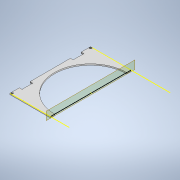
# Autodesk Inventor part: Box_Walls_2
Saved by Autodesk Inventor 2022 (Build 260153000, 153)
## iProperties
Created: 2023-02-27
Part Number: Box_Walls_2
Material: Generic
Document SubType Name: Modeling
Designer: zarek
Density: 1 g/cm^3
Appearance: Default
Author: zarek
Autodesk Inventor part; units mm, degrees
ref_plane "YZ Plane" through (0, 0, 0) normal (1, 0, 0) x (0, 1, 0)
ref_plane "XZ Plane" through (0, 0, 0) normal (0, 1, 0) x (-1, 0, 0)
ref_plane "XY Plane" through (0, 0, 0) normal (0, 0, 1) x (1, 0, 0)
sketch "Sketch1" plane through (0, 0, 0) normal (0, 1, 0) x (-1, 0, 0)
  line L0 (101.6, -101.6) -> (-101.6, -101.6)
  line L1 (-101.6, -101.6) -> (-101.6, 101.6)
  line L2 (-101.6, 101.6) -> (101.6, 101.6)
  line L3 (101.6, 101.6) -> (101.6, -101.6)
  line L4 (96.6, -96.6) -> (-96.6, -96.6)
  line L5 (-96.6, -96.6) -> (-96.6, 96.6)
  line L6 (-96.6, 96.6) -> (96.6, 96.6)
  line L7 (96.6, 96.6) -> (96.6, -96.6)
  line L8 (101.6, 101.6) -> (-40.4, 101.6)
  circle A0 centre (0, 0) radius 86.4
  circle A1 centre (0, 0) radius 109.3376
  line L9 (-40.4, 101.6) -> (-101.6, 40.4)
  line L10 (-45.4, 101.6) -> (-101.6, 45.4)
  line L11 (96.6, 96.6) -> (96.6, 101.6)
  line L12 (-45.4, 101.6) -> (-35.4, 101.6)
  line L13 (-35.4, 101.6) -> (-35.4, 96.6)
  line L14 (-35.4, 96.6) -> (-45.4, 96.6)
  line L15 (-45.4, 96.6) -> (-45.4, 101.6)
  circle A2 centre (0, 0) radius 111.3376
  point P0 (96.6, 51.2168)
  point P1 (101.6, 40.4)
  point P2 (101.6, -40.4)
  point P3 (96.6, -51.2168)
  point P4 (-96.6, 45.4)
  point P5 (-45.4, 96.6)
  dimension "d0" = 203.2
  dimension "d1" = 203.2
  dimension "d2" = 101.6
  dimension "d3" = 101.6
  dimension "d4" = 5
  dimension "d5" = 5
  dimension "d6" = 5
  dimension "d7" = 5
  dimension "d10" = 142
  dimension "d12" = 61.2
  dimension "d14" = 172.8
  dimension "d15" = 5
  dimension "d16" = 5
  dimension "d17" = 10
  dimension "d34" = 2
  constraints: 32 end point, 7 parallel, 6 point on line, 4 perpendicular, 3 centre point, 3 coincident, 3 horizontal, 2 point on circle
  measures "d0" distance between parallel lines of L2 L0
  measures "d1" distance between parallel lines of L1 L3
  measures "d2" distance from line of L0 point (0, 0)
  measures "d3" distance from line of L1 point (0, 0)
  measures "d4" distance between parallel lines of L4 L0
  measures "d5" distance between parallel lines of L1 L5
  measures "d6" distance between parallel lines of L2 L6
  measures "d7" distance between parallel lines of L3 L7
  measures "d10" distance of L2.end L8.end
  measures "d12" distance from line of L1 L8.end
  measures "d14" diameter of A0
  measures "d15" distance of L10.end L9.end
  measures "d16" distance of L10.start L8.end
  measures "d17" distance of L13.end L14.end
  measures "d34" radial gap between concentric circles of A1 A2
extrude "Extrusion1" add sketch "Sketch1" along normal blind 3 contours A2 L7 L4 | L4 A1 L7 A2 | L4 A1 L5 L9 L6 L7 | A2 L5 A1 L4 | L4 L5 A2 | A1 L6 A2 L7 | A2 L6 L7
sketch "Sketch5" plane through (0, 3, 0) normal (0, 1, 0) x (1, 0, 0)
  line L0 (-96.6, -96.6) -> (45.4, -96.6) projected
  circle A0 centre (0, 0) radius 86.4 projected
  line L1 (96.6, -45.4) -> (96.6, 96.6) projected
  line L2 (96.6, 0) -> (89.1, 0)
  line L3 (89.1, 0) -> (89.1, 10)
  line L4 (89.1, 10) -> (96.6, 10)
  line L5 (96.6, 10) -> (96.6, 0)
  line L6 (89.1, 0) -> (96.6, 0)
  line L7 (96.6, 0) -> (96.6, -10)
  line L8 (96.6, -10) -> (89.1, -10)
  line L9 (89.1, -10) -> (89.1, 0)
  line L10 (0, 0) -> (96.6, 0)
  point P0 (10, -96.6)
  dimension "d52" = 7.5
  dimension "d53" = 7.5
  dimension "d54" = 10
  dimension "d55" = 10
  constraints: 18 end point, 4 parallel, 3 horizontal, 2 perpendicular, 2 point on line
  measures "d52" distance of L3.end L4.end
  measures "d53" distance of L7.end L8.end
  measures "d54" distance between parallel lines of L6 L4
  measures "d55" distance between parallel lines of L10 L8
extrude "Extrusion4" add sketch "Sketch5" along normal blind 15 contours L3 L4 L1 L2 | L2 L1 L8 L9
sketch "Sketch7" plane through (89.1, 3, 10) normal (0, 0, 1) x (1, 0, 0)
  line L0 (2, 10) -> (5.5, 10)
  line L1 (5.5, 10) -> (5.5, 3)
  line L2 (5.5, 3) -> (2, 3)
  line L3 (2, 3) -> (2, 10)
  line L4 (7.5, 0) -> (7.5, 15)
  line L5 (0, 0) -> (0, 15)
  line L6 (0, 15) -> (7.5, 15)
  point P0 (-89.1, -3)
  dimension "d56" = 3.5
  dimension "d57" = 2
  dimension "d58" = 2
  dimension "d59" = 5
  dimension "d60" = 7
  constraints: 14 end point, 2 parallel, 1 horizontal, 1 perpendicular
  measures "d56" distance of L1.end L2.end
  measures "d57" distance between parallel lines of L4 L1
  measures "d58" distance between parallel lines of L5 L3
  measures "d59" distance between parallel lines of L0 L6
  measures "d60" distance between parallel lines of L2 L0
extrude "Extrusion6" cut sketch "Sketch7" against normal through all
fillet "Fillet7" radius 3.175 2 edges at (96.6, 18, 0) (89.1, 18, 0)
sketch "Sketch8" plane through (0, 3, 0) normal (0, 1, 0) x (1, 0, 0)
  arc A0 (-101.6, -98.425) -> (-98.425, -101.6) centre (-98.425, -98.425) ccw
  line L0 (44.0849, 101.6) -> (-98.425, 101.6)
  line L1 (-101.6, 98.425) -> (-101.6, -98.425)
  line L2 (-101.6, -46.1) -> (-101.6, -76.6)
  line L3 (-96.6, -96.6) -> (-96.6, 96.6)
  line L4 (-96.6, -46.1) -> (-96.6, -76.6)
  line L5 (-101.6, -76.6) -> (-96.6, -76.6)
  line L6 (-101.6, -46.1) -> (-96.6, -46.1)
  line L7 (-98.425, -101.6) -> (101.6, -101.6)
  line L8 (0, 0) -> (-101.6, 0)
  line L9 (-101.6, 46.1) -> (-101.6, 76.6)
  line L10 (-96.6, 46.1) -> (-96.6, 76.6)
  line L11 (-101.6, 76.6) -> (-96.6, 76.6)
  line L12 (-101.6, 46.1) -> (-96.6, 46.1)
  line L13 (-96.6, -76.6) -> (-90.1, -76.6)
  line L14 (-90.1, -76.6) -> (-90.1, -46.1)
  line L15 (-90.1, -46.1) -> (-96.6, -46.1)
  line L16 (-96.6, -46.1) -> (-96.6, -76.6)
  arc A1 (-98.425, 101.6) -> (-101.6, 98.425) centre (-98.425, 98.425) ccw
  line L17 (-101.6, 46.1) -> (-101.6, 76.6)
  line L18 (-96.6, 46.1) -> (-96.6, 76.6)
  line L19 (-101.6, 76.6) -> (-96.6, 76.6)
  line L20 (-101.6, 46.1) -> (-96.6, 46.1)
  line L21 (-96.6, 76.6) -> (-90.1, 76.6)
  line L22 (-90.1, 76.6) -> (-90.1, 46.1)
  line L23 (-90.1, 46.1) -> (-96.6, 46.1)
  line L24 (-96.6, 46.1) -> (-96.6, 76.6)
  line L25 (-96.6, -76.6) -> (-101.6, -76.6)
  line L26 (-101.6, -76.6) -> (-101.6, -74.1)
  line L27 (-101.6, -74.1) -> (-96.6, -74.1)
  line L28 (-96.6, -74.1) -> (-96.6, -76.6)
  line L29 (-96.6, -46.1) -> (-101.6, -46.1)
  line L30 (-101.6, -46.1) -> (-101.6, -48.6)
  line L31 (-101.6, -48.6) -> (-96.6, -48.6)
  line L32 (-96.6, -48.6) -> (-96.6, -46.1)
  line L33 (-96.6, -76.6) -> (-90.1, -76.6)
  line L34 (-90.1, -76.6) -> (-90.1, -74.1)
  line L35 (-90.1, -74.1) -> (-96.6, -74.1)
  line L36 (-96.6, -74.1) -> (-96.6, -76.6)
  line L37 (-96.6, -48.6) -> (-90.1, -48.6)
  line L38 (-90.1, -48.6) -> (-90.1, -46.1)
  line L39 (-90.1, -46.1) -> (-96.6, -46.1)
  line L40 (-96.6, -46.1) -> (-96.6, -48.6)
  line L41 (-96.6, 96.6) -> (-96.6, -96.6) projected
  line L42 (-90.1, 46.1) -> (-96.6, 46.1)
  line L43 (-96.6, 46.1) -> (-96.6, 48.6)
  line L44 (-96.6, 48.6) -> (-90.1, 48.6)
  line L45 (-90.1, 48.6) -> (-90.1, 46.1)
  line L46 (-90.1, 76.6) -> (-96.6, 76.6)
  line L47 (-96.6, 76.6) -> (-96.6, 74.1)
  line L48 (-96.6, 74.1) -> (-90.1, 74.1)
  line L49 (-90.1, 74.1) -> (-90.1, 76.6)
  point P0 (-98.425, 98.425)
  point P1 (46.1, 101.6)
  point P2 (46.1, 96.6)
  point P3 (76.6, 96.6)
  point P4 (76.6, 101.6)
  point P5 (-46.1, 96.6)
  dimension "d64" = 30.5
  dimension "d65" = 25
  dimension "d66" = 6.5
  dimension "d118" = 2.5
  dimension "d119" = 2.5
  dimension "d120" = 2.5
  dimension "d121" = 2.5
  constraints: 98 end point, 15 parallel, 10 symmetric about line, 8 perpendicular, 7 horizontal, 6 point on line, 4 point on circle, 2 centre point, 1 midpoint, 4 other
  measures "d64" distance between parallel lines of L5 L6
  measures "d65" distance between parallel lines of L5 L7
  measures "d66" distance between parallel lines of L14 L3
  measures "d118" distance of L25.end L26.end
  measures "d119" distance of L30.end L29.end
  measures "d120" distance of L42.end L43.end
  measures "d121" distance of L47.end L46.end
extrude "Extrusion7" cut sketch "Sketch8" against normal through all contours L48 L22 L44 L3 | L37 L14 L35 L3
sketch "Sketch11" plane through (0, 3, 0) normal (0, 1, 0) x (1, 0, 0)
  line L0 (-94, 94) -> (94, 94)
  line L1 (94, 94) -> (94, -94)
  line L2 (94, -94) -> (-94, -94)
  line L3 (-94, -94) -> (-94, 94)
  circle A0 centre (-94, 94) radius 1.5
  circle A1 centre (94, 94) radius 1.5
  circle A2 centre (-94, -94) radius 1.5
  circle A3 centre (94, -39.0849) radius 1.5
  point P0 (0, 0)
  point P1 (0, 0)
  dimension "d98" = 94
  dimension "d99" = 94
  dimension "d100" = 94
  dimension "d101" = 94
  dimension "d102" = 3
  dimension "d103" = 3
  dimension "d104" = 3
  dimension "d105" = 3
  constraints: 8 end point, 4 centre point, 3 coincident, 2 parallel, 1 horizontal, 1 perpendicular, 1 point on line
  measures "d98" distance from line of point (0, 0) L0
  measures "d99" distance from line of point (0, 0) L3
  measures "d100" distance from line of point (0, 0) L1
  measures "d101" distance from line of L2 point (0, 0)
  measures "d102" diameter of A0
  measures "d103" diameter of A1
  measures "d104" diameter of A2
  measures "d105" diameter of A3
extrude "Extrusion8" cut sketch "Sketch11" against normal blind 10 contours L3 A0 L0 | L0 A0 L3 | A1 L1 L0 | L0 L1 A1 | A2 L2 L3 | L3 L2 A2 | A3 L1 | L1 A3
sketch "Sketch12" plane through (0, 3, 0) normal (0, 1, 0) x (1, 0, 0)
  line L0 (-94, 94) -> (94, 94)
  line L1 (94, 94) -> (94, -94)
  line L2 (94, -94) -> (-94, -94)
  line L3 (-94, -94) -> (-94, 94)
  circle A0 centre (-94, 94) radius 2.6
  circle A1 centre (94, 94) radius 2.6
  circle A2 centre (-94, -94) radius 2.6
  circle A3 centre (94, -39.0849) radius 2.6
  point P0 (0, 0)
  point P1 (0, 0)
  point P2 (0, 0)
  dimension "d108" = 94
  dimension "d109" = 94
  dimension "d110" = 94
  dimension "d111" = 94
  dimension "d112" = 5.2
  dimension "d113" = 5.2
  dimension "d114" = 5.2
  dimension "d115" = 5.2
  constraints: 8 end point, 4 centre point, 3 coincident, 2 parallel, 1 horizontal, 1 perpendicular, 1 point on line
  measures "d108" distance from line of point (0, 0) L0
  measures "d109" distance from line of point (0, 0) L3
  measures "d110" distance from line of point (0, 0) L1
  measures "d111" distance from line of L2 point (0, 0)
  measures "d112" diameter of A0
  measures "d113" diameter of A1
  measures "d114" diameter of A2
  measures "d115" diameter of A3
extrude "Extrusion9" cut sketch "Sketch12" against normal blind 1.5 contours L3 A0 L0 | L0 A0 L3 | A1 L1 L0 | L0 L1 A1 | A2 L2 L3 | L3 L2 A2 | A3 L1 | L1 A3
sketch "Sketch13" plane through (0, 3, 0) normal (0, 1, 0) x (1, 0, 0)
  line L0 (94, 96.6) -> (-94, 96.6) projected
  line L1 (0, 96.6) -> (0, -96.6)
  line L2 (-96.6, -96.6) -> (45.4, -96.6) projected
  point P0 (0, 0)
  constraints: 2 end point, 1 midpoint, 1 point on line, 1 vertical
ref_plane "Work Plane1" through (0, 3, -96.6) normal (-1, 0, 0) x (0, 0, 1)
sketch "Sketch14" plane through (0, 3, -96.6) normal (-1, 0, 0) x (0, 0, 1)
  line L0 (208.9015, 36.251) -> (-17.5186, 36.251)
  line L1 (-17.5186, 36.251) -> (-17.5186, -18.9911)
  line L2 (-17.5186, -18.9911) -> (208.9015, -18.9911)
  line L3 (208.9015, -18.9911) -> (208.9015, 36.251)
  point P0 (96.6, -3)
  constraints: 8 end point, 2 parallel, 1 horizontal, 1 perpendicular
extrude "Extrusion10" cut sketch "Sketch14" against normal through all
sketch "Sketch15" plane through (-96.6, 0, -48.6) normal (-1, 0, 0) x (0, 0, 1)
  line L0 (-43.9, 0) -> (-46.9, 0) projected
  line L1 (141.1, 1.5) -> (141.1, 0) projected
  line L2 (-43.9, 0) -> (141.1, 0)
  line L3 (141.1, 0) -> (141.1, 1)
  line L4 (141.1, 1) -> (-43.9, 1)
  line L5 (-43.9, 1) -> (-43.9, 0)
  point P0 (48.6, 0)
  dimension "d125" = 1
  constraints: 8 end point, 2 parallel, 1 horizontal, 1 perpendicular, 1 point on line
  measures "d125" distance of L3.end L2.end
extrude "Extrusion11" cut sketch "Sketch15" against normal blind 1
equation "\"d1\" = d0"
equation "\"d2\" = 0.5 * d0"
equation "\"d3\" = 0.5 * d0"
body "Solid1"
